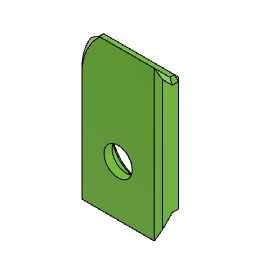
Magnet_Mount_Lid_M2 (Autodesk Fusion 360 design; units mm, degrees)
Autodesk Fusion 360 part; units mm, degrees
sketch "Skizze1" plane through (0, 0, 0) normal (1, 0, 0) x (0, 1, 0)
  line L0 (0, 0) -> (0, 7.5)
  line L1 (0, 7.5) -> (-1, 7.5) construction
  line L2 (-1, 7.5) -> (-3, 9.5) construction
  line L3 (-3, 9.5) -> (-3, 0)
  line L4 (0, 0) -> (-3, 0)
  line L5 (0, 0) -> (0, -7.5)
  line L6 (0, -7.5) -> (-1, -7.5) construction
  line L7 (-1, -7.5) -> (-3, -9.5) construction
  line L8 (-3, -9.5) -> (-3, 0)
  line L9 (0, 7.35) -> (-1.0621, 7.35)
  line L10 (-1.0621, 7.35) -> (-3, 9.2879)
  line L11 (0, -7.35) -> (-1.0621, -7.35)
  line L12 (-1.0621, -7.35) -> (-3, -9.2879)
  dimension "d24" = 135
  dimension "d25" = 7.5
  dimension "d26" = 2
  dimension "d27" = 1
  dimension "d28" = 0.15
  dimension "d29" = 0.15
  constraint coincident L0.start L4.start
  constraint vertical L0
  constraint perpendicular L0 L1
  constraint vertical L3
  constraint perpendicular L3 L4
  constraint symmetric L0.start L4 L5.start
  constraint symmetric L0.end L4 L5.end
  constraint symmetric L1.end L4 L6.end
  constraint symmetric L2.end L4 L7.end
  constraint symmetric L3.end L4 L8.end
  constraint coincident L0 L9.start
  constraint perpendicular L0 L9
  constraint coincident L3 L10.end
  constraint parallel L2 L10
  constraint symmetric L4 L9.start L11.start
  constraint symmetric L4 L9.end L11.end
  constraint symmetric L4 L10.end L12.end
  measures "d24" angle of L1 L2
  measures "d25" distance of L0.start L0.end
  measures "d26" vertical distance of L1.end L2.end
  measures "d27" distance of L0.end L1.end
  measures "d28" distance of L1 L9
  measures "d29" distance of L2 L10
extrude "Extrusion1" add sketch "Skizze1" along normal mid plane 10
sketch "Skizze2" plane through (0, 0, 0) normal (0, 1, 0) x (-1, 0, 0)
  line L0 (5, 7.35) -> (-5, 7.35)
  line L1 (-5, -7.35) -> (5, -7.35)
  line L2 (-5, 7.35) -> (-5, -7.35)
  line L3 (5, -7.35) -> (5, 7.35)
  point P0 (0, -3)
  dimension "d44" = 4.35
  constraint vertical origin P0
  measures "d44" distance of L1 P0
hole "Bohrung1" at (0, 0, -3) direction (0, -1, 0) diameter 3.5 end up to surface (3 mm away) counterbore diameter 6.5 counterbore depth 2
sketch "Skizze3" plane through (0, -3, 0) normal (0, -1, 0) x (1, 0, 0)
  circle A0 centre (0, -3) radius 1.75
  line L0 (-5, -9.2879) -> (5, -9.2879)
  line L1 (5, -9.2879) -> (5, 9.2879)
  line L2 (5, 9.2879) -> (-5, 9.2879)
  line L3 (-5, 9.2879) -> (-5, -9.2879)
  arc A1 (-1.3196, 10.5604) -> (-5, 4.25) centre (2.25, 4.25) ccw
  arc A2 (2.25, 11.5) -> (-5, 4.25) centre (2.25, 4.25) ccw
  arc A3 (2.25, 11.5) -> (-3.8568, 8.1576) centre (2.25, 4.25) ccw
  spline S0 degree 3 poles (-1.3196, 10.5604) (-1.7097, 10.3397) (-2.082, 10.0811) (-2.7755, 9.4953) (-3.0966, 9.168) (-3.385, 8.8117) (-3.5136, 8.6529) (-3.6357, 8.4883) (-3.7868, 8.2654) (-3.8222, 8.2117) (-3.8568, 8.1576) knots -2.594988 -2.594988 -2.594988 -2.594988 -2.401547 -2.401547 -2.208106 -2.208106 -2.208106 -2.121869 -2.121869 -2.094868 -2.094868 -2.094868 -2.094868
  line L4 (-5, -10.7071) -> (-5, -8.2071)
  line L5 (-5, -8.2071) -> (-5, -15.45)
  line L6 (-5, -15.45) -> (-5, 4.25)
  line L7 (-5, 4.25) -> (-5, -10.7071)
extrude "Extrusion2" cut sketch "Skizze3" against normal through all contours L2 L3 A1 A2 A3 S0
chamfer "Fase1" distance 0.5 angle 45 16 edges at (5, -3, 0) (5, -2.0311, 8.3189) (5, -0.5311, 7.35) (5, 0, 0) (5, -0.5311, -7.35) (5, -2.0311, -8.3189) (-5, -3, -2.5189) (-4.4717, -3, 6.9669) (-5, 0, -1.55) (-4.8238, 0, 5.8386) (-5, -0.5311, -7.35) (-5, -2.0311, -8.3189) (0, 0, -7.35) (0.3481, 0, 7.35) (-3.713, -2.0859, 8.3737) (1.1753, 0, -6.0301)
equation "d25 = ( 15 / 2 ) * 1 mm"
equation "d29 = d28"
equation "d44 = 4.5 mm - 0.15 mm"
named bodies: "Magnet_Mount_Lid"
